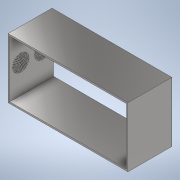
# Autodesk Inventor part: corpo-meio
Saved by Autodesk Inventor 2021 (Build 250183000, 183)
## iProperties
Created: 2023-11-09
Part Number: corpo-meio
Material: Genérico
Document SubType Name: Modeling
Designer: Vinicius
Density: 1 g/cm^3
Appearance: Padrão
Author: Vinicius
Autodesk Inventor part; units mm, degrees
ref_plane "YZ Plane" through (0, 0, 0) normal (1, 0, 0) x (0, 1, 0)
ref_plane "XZ Plane" through (0, 0, 0) normal (0, 1, 0) x (-1, 0, 0)
ref_plane "XY Plane" through (0, 0, 0) normal (0, 0, 1) x (1, 0, 0)
sketch "Esboço2" plane through (0, 0, 0) normal (0, 0, 1) x (1, 0, 0)
  line L0 (-300, -150) -> (300, -150)
  line L1 (300, -150) -> (300, 150)
  line L2 (300, 150) -> (-300, 150)
  line L3 (-300, 150) -> (-300, -150)
  line L4 (-300, -150) -> (300, 150) construction
  line L5 (300, -150) -> (-300, 150) construction
  line L6 (-292, -142) -> (292, -142)
  line L7 (292, -142) -> (292, 142)
  line L8 (292, 142) -> (-292, 142)
  line L9 (-292, 142) -> (-292, -142)
  line L10 (-292, -142) -> (292, 142) construction
  line L11 (292, -142) -> (-292, 142) construction
  point P0 (0, 0)
  dimension "d0" = 300
  dimension "d1" = 600
  dimension "d2" = 584
  dimension "d3" = 284
  constraints: 24 end point, 4 midpoint, 4 parallel, 2 horizontal, 2 perpendicular
  measures "d0" distance of L2.end L0.start
  measures "d1" distance of L1.end L2.end
  measures "d2" distance of L8.end L7.end
  measures "d3" distance of L8.end L6.start
extrude "Extrusão1" add sketch "Esboço2" along normal blind 220
sketch "Esboço3" plane through (-300, -150, 0) normal (-1, 0, 0) x (0, 0, 1)
  line L0 (220, 8) -> (220, 292) projected
  line L1 (0, 0) -> (220, 0) projected
  line L2 (0, 292) -> (220, 292) projected
  line L3 (165, 150) -> (125, 150)
  circle A0 centre (165, 150) radius 1.5
  circle A1 centre (160, 150) radius 1.5
  circle A2 centre (155, 150) radius 1.5
  circle A3 centre (150, 150) radius 1.5
  circle A4 centre (145, 150) radius 1.5
  circle A5 centre (140, 150) radius 1.5
  circle A6 centre (135, 150) radius 1.5
  circle A7 centre (130, 150) radius 1.5
  circle A8 centre (125, 150) radius 1.5
  circle A9 centre (163.4549, 145.2447) radius 1.5
  circle A10 centre (169.0451, 147.0611) radius 1.5
  circle A11 centre (169.0451, 152.9389) radius 1.5
  circle A12 centre (163.4549, 154.7553) radius 1.5
  circle A13 centre (156.9098, 144.1221) radius 1.5
  circle A14 centre (161.9098, 140.4894) radius 1.5
  circle A15 centre (168.0902, 140.4894) radius 1.5
  circle A16 centre (173.0902, 144.1221) radius 1.5
  circle A17 centre (175, 150) radius 1.5
  circle A18 centre (173.0902, 155.8779) radius 1.5
  circle A19 centre (168.0902, 159.5106) radius 1.5
  circle A20 centre (161.9098, 159.5106) radius 1.5
  circle A21 centre (156.9098, 155.8779) radius 1.5
  circle A22 centre (151.2968, 143.899) radius 1.5
  circle A23 centre (154.963, 138.8528) radius 1.5
  circle A24 centre (160.3647, 135.7342) radius 1.5
  circle A25 centre (166.5679, 135.0822) radius 1.5
  circle A26 centre (172.5, 137.0096) radius 1.5
  circle A27 centre (177.1353, 141.1832) radius 1.5
  circle A28 centre (179.6722, 146.8813) radius 1.5
  circle A29 centre (179.6722, 153.1187) radius 1.5
  circle A30 centre (177.1353, 158.8168) radius 1.5
  circle A31 centre (172.5, 162.9904) radius 1.5
  circle A32 centre (166.5679, 164.9178) radius 1.5
  circle A33 centre (160.3647, 164.2658) radius 1.5
  circle A34 centre (154.963, 161.1472) radius 1.5
  circle A35 centre (151.2968, 156.101) radius 1.5
  circle A36 centre (145.9789, 143.8197) radius 1.5
  circle A37 centre (148.8197, 138.2443) radius 1.5
  circle A38 centre (153.2443, 133.8197) radius 1.5
  circle A39 centre (158.8197, 130.9789) radius 1.5
  circle A40 centre (165, 130) radius 1.5
  circle A41 centre (171.1803, 130.9789) radius 1.5
  circle A42 centre (176.7557, 133.8197) radius 1.5
  circle A43 centre (181.1803, 138.2443) radius 1.5
  circle A44 centre (184.0211, 143.8197) radius 1.5
  circle A45 centre (185, 150) radius 1.5
  circle A46 centre (184.0211, 156.1803) radius 1.5
  circle A47 centre (181.1803, 161.7557) radius 1.5
  circle A48 centre (176.7557, 166.1803) radius 1.5
  circle A49 centre (171.1803, 169.0211) radius 1.5
  circle A50 centre (165, 170) radius 1.5
  circle A51 centre (158.8197, 169.0211) radius 1.5
  circle A52 centre (153.2443, 166.1803) radius 1.5
  circle A53 centre (148.8197, 161.7557) radius 1.5
  circle A54 centre (145.9789, 156.1803) radius 1.5
  circle A55 centre (140.7854, 143.7828) radius 1.5
  circle A56 centre (143.0923, 137.9562) radius 1.5
  circle A57 centre (146.7758, 132.8863) radius 1.5
  circle A58 centre (151.6043, 128.8918) radius 1.5
  circle A59 centre (157.2746, 126.2236) radius 1.5
  circle A60 centre (163.4302, 125.0493) radius 1.5
  circle A61 centre (169.6845, 125.4428) radius 1.5
  circle A62 centre (175.6445, 127.3793) radius 1.5
  circle A63 centre (180.9356, 130.7372) radius 1.5
  circle A64 centre (185.2254, 135.3054) radius 1.5
  circle A65 centre (188.2444, 140.7969) radius 1.5
  circle A66 centre (189.8029, 146.8667) radius 1.5
  circle A67 centre (189.8029, 153.1333) radius 1.5
  circle A68 centre (188.2444, 159.2031) radius 1.5
  circle A69 centre (185.2254, 164.6946) radius 1.5
  circle A70 centre (180.9356, 169.2628) radius 1.5
  circle A71 centre (175.6445, 172.6207) radius 1.5
  circle A72 centre (169.6845, 174.5572) radius 1.5
  circle A73 centre (163.4302, 174.9507) radius 1.5
  circle A74 centre (157.2746, 173.7764) radius 1.5
  circle A75 centre (151.6043, 171.1082) radius 1.5
  circle A76 centre (146.7758, 167.1137) radius 1.5
  circle A77 centre (143.0923, 162.0438) radius 1.5
  circle A78 centre (140.7854, 156.2172) radius 1.5
  circle A79 centre (135.6556, 143.7626) radius 1.5
  circle A80 centre (137.5936, 137.7979) radius 1.5
  circle A81 centre (140.7295, 132.3664) radius 1.5
  circle A82 centre (144.9261, 127.7057) radius 1.5
  circle A83 centre (150, 124.0192) radius 1.5
  circle A84 centre (155.7295, 121.4683) radius 1.5
  circle A85 centre (161.8641, 120.1643) radius 1.5
  circle A86 centre (168.1359, 120.1643) radius 1.5
  circle A87 centre (174.2705, 121.4683) radius 1.5
  circle A88 centre (180, 124.0192) radius 1.5
  circle A89 centre (185.0739, 127.7057) radius 1.5
  circle A90 centre (189.2705, 132.3664) radius 1.5
  circle A91 centre (192.4064, 137.7979) radius 1.5
  circle A92 centre (194.3444, 143.7626) radius 1.5
  circle A93 centre (195, 150) radius 1.5
  circle A94 centre (194.3444, 156.2374) radius 1.5
  circle A95 centre (192.4064, 162.2021) radius 1.5
  circle A96 centre (189.2705, 167.6336) radius 1.5
  circle A97 centre (185.0739, 172.2943) radius 1.5
  circle A98 centre (180, 175.9808) radius 1.5
  circle A99 centre (174.2705, 178.5317) radius 1.5
  circle A100 centre (168.1359, 179.8357) radius 1.5
  circle A101 centre (161.8641, 179.8357) radius 1.5
  circle A102 centre (155.7295, 178.5317) radius 1.5
  circle A103 centre (150, 175.9808) radius 1.5
  circle A104 centre (144.9261, 172.2943) radius 1.5
  circle A105 centre (140.7295, 167.6336) radius 1.5
  circle A106 centre (137.5936, 162.2021) radius 1.5
  circle A107 centre (135.6556, 156.2374) radius 1.5
  circle A108 centre (130.5625, 143.7505) radius 1.5
  circle A109 centre (132.2318, 137.7019) radius 1.5
  circle A110 centre (134.9543, 132.0485) radius 1.5
  circle A111 centre (138.6425, 126.9721) radius 1.5
  circle A112 centre (143.1779, 122.6359) radius 1.5
  circle A113 centre (148.4146, 119.1792) radius 1.5
  circle A114 centre (154.1844, 116.713) radius 1.5
  circle A115 centre (160.3018, 115.3168) radius 1.5
  circle A116 centre (166.5703, 115.0352) radius 1.5
  circle A117 centre (172.7882, 115.8775) radius 1.5
  circle A118 centre (178.7559, 117.8165) radius 1.5
  circle A119 centre (184.2814, 120.7899) radius 1.5
  circle A120 centre (189.1872, 124.7022) radius 1.5
  circle A121 centre (193.3156, 129.4275) radius 1.5
  circle A122 centre (196.5339, 134.8141) radius 1.5
  circle A123 centre (198.7387, 140.6887) radius 1.5
  circle A124 centre (199.8591, 146.8626) radius 1.5
  circle A125 centre (199.8591, 153.1374) radius 1.5
  circle A126 centre (198.7387, 159.3113) radius 1.5
  circle A127 centre (196.5339, 165.1859) radius 1.5
  circle A128 centre (193.3156, 170.5725) radius 1.5
  circle A129 centre (189.1872, 175.2978) radius 1.5
  circle A130 centre (184.2814, 179.2101) radius 1.5
  circle A131 centre (178.7559, 182.1835) radius 1.5
  circle A132 centre (172.7882, 184.1225) radius 1.5
  circle A133 centre (166.5703, 184.9648) radius 1.5
  circle A134 centre (160.3018, 184.6832) radius 1.5
  circle A135 centre (154.1844, 183.287) radius 1.5
  circle A136 centre (148.4146, 180.8208) radius 1.5
  circle A137 centre (143.1779, 177.3641) radius 1.5
  circle A138 centre (138.6425, 173.0279) radius 1.5
  circle A139 centre (134.9543, 167.9515) radius 1.5
  circle A140 centre (132.2318, 162.2981) radius 1.5
  circle A141 centre (130.5625, 156.2495) radius 1.5
  circle A142 centre (125.4925, 143.7426) radius 1.5
  circle A143 centre (126.9577, 137.6393) radius 1.5
  circle A144 centre (129.3597, 131.8404) radius 1.5
  circle A145 centre (132.6393, 126.4886) radius 1.5
  circle A146 centre (136.7157, 121.7157) radius 1.5
  circle A147 centre (141.4886, 117.6393) radius 1.5
  circle A148 centre (146.8404, 114.3597) radius 1.5
  circle A149 centre (152.6393, 111.9577) radius 1.5
  circle A150 centre (158.7426, 110.4925) radius 1.5
  circle A151 centre (165, 110) radius 1.5
  circle A152 centre (171.2574, 110.4925) radius 1.5
  circle A153 centre (177.3607, 111.9577) radius 1.5
  circle A154 centre (183.1596, 114.3597) radius 1.5
  circle A155 centre (188.5114, 117.6393) radius 1.5
  circle A156 centre (193.2843, 121.7157) radius 1.5
  circle A157 centre (197.3607, 126.4886) radius 1.5
  circle A158 centre (200.6403, 131.8404) radius 1.5
  circle A159 centre (203.0423, 137.6393) radius 1.5
  circle A160 centre (204.5075, 143.7426) radius 1.5
  circle A161 centre (205, 150) radius 1.5
  circle A162 centre (204.5075, 156.2574) radius 1.5
  circle A163 centre (203.0423, 162.3607) radius 1.5
  circle A164 centre (200.6403, 168.1596) radius 1.5
  circle A165 centre (197.3607, 173.5114) radius 1.5
  circle A166 centre (193.2843, 178.2843) radius 1.5
  circle A167 centre (188.5114, 182.3607) radius 1.5
  circle A168 centre (183.1596, 185.6403) radius 1.5
  circle A169 centre (177.3607, 188.0423) radius 1.5
  circle A170 centre (171.2574, 189.5075) radius 1.5
  circle A171 centre (165, 190) radius 1.5
  circle A172 centre (158.7426, 189.5075) radius 1.5
  circle A173 centre (152.6393, 188.0423) radius 1.5
  circle A174 centre (146.8404, 185.6403) radius 1.5
  circle A175 centre (141.4886, 182.3607) radius 1.5
  circle A176 centre (136.7157, 178.2843) radius 1.5
  circle A177 centre (132.6393, 173.5114) radius 1.5
  circle A178 centre (129.3597, 168.1596) radius 1.5
  circle A179 centre (126.9577, 162.3607) radius 1.5
  circle A180 centre (125.4925, 156.2574) radius 1.5
  line L4 (0, 8) -> (0, 292)
  circle A181 centre (55, 150) radius 1.5
  circle A182 centre (60, 150) radius 1.5
  circle A183 centre (65, 150) radius 1.5
  circle A184 centre (70, 150) radius 1.5
  circle A185 centre (75, 150) radius 1.5
  circle A186 centre (80, 150) radius 1.5
  circle A187 centre (85, 150) radius 1.5
  circle A188 centre (90, 150) radius 1.5
  circle A189 centre (95, 150) radius 1.5
  circle A190 centre (56.5451, 145.2447) radius 1.5
  circle A191 centre (50.9549, 147.0611) radius 1.5
  circle A192 centre (50.9549, 152.9389) radius 1.5
  circle A193 centre (56.5451, 154.7553) radius 1.5
  circle A194 centre (63.0902, 144.1221) radius 1.5
  circle A195 centre (58.0902, 140.4894) radius 1.5
  circle A196 centre (51.9098, 140.4894) radius 1.5
  circle A197 centre (46.9098, 144.1221) radius 1.5
  circle A198 centre (45, 150) radius 1.5
  circle A199 centre (46.9098, 155.8779) radius 1.5
  circle A200 centre (51.9098, 159.5106) radius 1.5
  circle A201 centre (58.0902, 159.5106) radius 1.5
  circle A202 centre (63.0902, 155.8779) radius 1.5
  circle A203 centre (68.7032, 143.899) radius 1.5
  circle A204 centre (65.037, 138.8528) radius 1.5
  circle A205 centre (59.6353, 135.7342) radius 1.5
  circle A206 centre (53.4321, 135.0822) radius 1.5
  circle A207 centre (47.5, 137.0096) radius 1.5
  circle A208 centre (42.8647, 141.1832) radius 1.5
  circle A209 centre (40.3278, 146.8813) radius 1.5
  circle A210 centre (40.3278, 153.1187) radius 1.5
  circle A211 centre (42.8647, 158.8168) radius 1.5
  circle A212 centre (47.5, 162.9904) radius 1.5
  circle A213 centre (53.4321, 164.9178) radius 1.5
  circle A214 centre (59.6353, 164.2658) radius 1.5
  circle A215 centre (65.037, 161.1472) radius 1.5
  circle A216 centre (68.7032, 156.101) radius 1.5
  circle A217 centre (74.0211, 143.8197) radius 1.5
  circle A218 centre (71.1803, 138.2443) radius 1.5
  circle A219 centre (66.7557, 133.8197) radius 1.5
  circle A220 centre (61.1803, 130.9789) radius 1.5
  circle A221 centre (55, 130) radius 1.5
  circle A222 centre (48.8197, 130.9789) radius 1.5
  circle A223 centre (43.2443, 133.8197) radius 1.5
  circle A224 centre (38.8197, 138.2443) radius 1.5
  circle A225 centre (35.9789, 143.8197) radius 1.5
  circle A226 centre (35, 150) radius 1.5
  circle A227 centre (35.9789, 156.1803) radius 1.5
  circle A228 centre (38.8197, 161.7557) radius 1.5
  circle A229 centre (43.2443, 166.1803) radius 1.5
  circle A230 centre (48.8197, 169.0211) radius 1.5
  circle A231 centre (55, 170) radius 1.5
  circle A232 centre (61.1803, 169.0211) radius 1.5
  circle A233 centre (66.7557, 166.1803) radius 1.5
  circle A234 centre (71.1803, 161.7557) radius 1.5
  circle A235 centre (74.0211, 156.1803) radius 1.5
  circle A236 centre (79.2146, 143.7828) radius 1.5
  circle A237 centre (76.9077, 137.9562) radius 1.5
  circle A238 centre (73.2242, 132.8863) radius 1.5
  circle A239 centre (68.3957, 128.8918) radius 1.5
  circle A240 centre (62.7254, 126.2236) radius 1.5
  circle A241 centre (56.5698, 125.0493) radius 1.5
  circle A242 centre (50.3155, 125.4428) radius 1.5
  circle A243 centre (44.3555, 127.3793) radius 1.5
  circle A244 centre (39.0644, 130.7372) radius 1.5
  circle A245 centre (34.7746, 135.3054) radius 1.5
  circle A246 centre (31.7556, 140.7969) radius 1.5
  circle A247 centre (30.1971, 146.8667) radius 1.5
  circle A248 centre (30.1971, 153.1333) radius 1.5
  circle A249 centre (31.7556, 159.2031) radius 1.5
  circle A250 centre (34.7746, 164.6946) radius 1.5
  circle A251 centre (39.0644, 169.2628) radius 1.5
  circle A252 centre (44.3555, 172.6207) radius 1.5
  circle A253 centre (50.3155, 174.5572) radius 1.5
  circle A254 centre (56.5698, 174.9507) radius 1.5
  circle A255 centre (62.7254, 173.7764) radius 1.5
  circle A256 centre (68.3957, 171.1082) radius 1.5
  circle A257 centre (73.2242, 167.1137) radius 1.5
  circle A258 centre (76.9077, 162.0438) radius 1.5
  circle A259 centre (79.2146, 156.2172) radius 1.5
  circle A260 centre (84.3444, 143.7626) radius 1.5
  circle A261 centre (82.4064, 137.7979) radius 1.5
  circle A262 centre (79.2705, 132.3664) radius 1.5
  circle A263 centre (75.0739, 127.7057) radius 1.5
  circle A264 centre (70, 124.0192) radius 1.5
  circle A265 centre (64.2705, 121.4683) radius 1.5
  circle A266 centre (58.1359, 120.1643) radius 1.5
  circle A267 centre (51.8641, 120.1643) radius 1.5
  circle A268 centre (45.7295, 121.4683) radius 1.5
  circle A269 centre (40, 124.0192) radius 1.5
  circle A270 centre (34.9261, 127.7057) radius 1.5
  circle A271 centre (30.7295, 132.3664) radius 1.5
  circle A272 centre (27.5936, 137.7979) radius 1.5
  circle A273 centre (25.6556, 143.7626) radius 1.5
  circle A274 centre (25, 150) radius 1.5
  circle A275 centre (25.6556, 156.2374) radius 1.5
  circle A276 centre (27.5936, 162.2021) radius 1.5
  circle A277 centre (30.7295, 167.6336) radius 1.5
  circle A278 centre (34.9261, 172.2943) radius 1.5
  circle A279 centre (40, 175.9808) radius 1.5
  circle A280 centre (45.7295, 178.5317) radius 1.5
  circle A281 centre (51.8641, 179.8357) radius 1.5
  circle A282 centre (58.1359, 179.8357) radius 1.5
  circle A283 centre (64.2705, 178.5317) radius 1.5
  circle A284 centre (70, 175.9808) radius 1.5
  circle A285 centre (75.0739, 172.2943) radius 1.5
  circle A286 centre (79.2705, 167.6336) radius 1.5
  circle A287 centre (82.4064, 162.2021) radius 1.5
  circle A288 centre (84.3444, 156.2374) radius 1.5
  circle A289 centre (89.4375, 143.7505) radius 1.5
  circle A290 centre (87.7682, 137.7019) radius 1.5
  circle A291 centre (85.0457, 132.0485) radius 1.5
  circle A292 centre (81.3575, 126.9721) radius 1.5
  circle A293 centre (76.8221, 122.6359) radius 1.5
  circle A294 centre (71.5854, 119.1792) radius 1.5
  circle A295 centre (65.8156, 116.713) radius 1.5
  circle A296 centre (59.6982, 115.3168) radius 1.5
  circle A297 centre (53.4297, 115.0352) radius 1.5
  circle A298 centre (47.2118, 115.8775) radius 1.5
  circle A299 centre (41.2441, 117.8165) radius 1.5
  circle A300 centre (35.7186, 120.7899) radius 1.5
  circle A301 centre (30.8128, 124.7022) radius 1.5
  circle A302 centre (26.6844, 129.4275) radius 1.5
  circle A303 centre (23.4661, 134.8141) radius 1.5
  circle A304 centre (21.2613, 140.6887) radius 1.5
  circle A305 centre (20.1409, 146.8626) radius 1.5
  circle A306 centre (20.1409, 153.1374) radius 1.5
  circle A307 centre (21.2613, 159.3113) radius 1.5
  circle A308 centre (23.4661, 165.1859) radius 1.5
  circle A309 centre (26.6844, 170.5725) radius 1.5
  circle A310 centre (30.8128, 175.2978) radius 1.5
  circle A311 centre (35.7186, 179.2101) radius 1.5
  circle A312 centre (41.2441, 182.1835) radius 1.5
  circle A313 centre (47.2118, 184.1225) radius 1.5
  circle A314 centre (53.4297, 184.9648) radius 1.5
  circle A315 centre (59.6982, 184.6832) radius 1.5
  circle A316 centre (65.8156, 183.287) radius 1.5
  circle A317 centre (71.5854, 180.8208) radius 1.5
  circle A318 centre (76.8221, 177.3641) radius 1.5
  circle A319 centre (81.3575, 173.0279) radius 1.5
  circle A320 centre (85.0457, 167.9515) radius 1.5
  circle A321 centre (87.7682, 162.2981) radius 1.5
  circle A322 centre (89.4375, 156.2495) radius 1.5
  circle A323 centre (94.5075, 143.7426) radius 1.5
  circle A324 centre (93.0423, 137.6393) radius 1.5
  circle A325 centre (90.6403, 131.8404) radius 1.5
  circle A326 centre (87.3607, 126.4886) radius 1.5
  circle A327 centre (83.2843, 121.7157) radius 1.5
  circle A328 centre (78.5114, 117.6393) radius 1.5
  circle A329 centre (73.1596, 114.3597) radius 1.5
  circle A330 centre (67.3607, 111.9577) radius 1.5
  circle A331 centre (61.2574, 110.4925) radius 1.5
  circle A332 centre (55, 110) radius 1.5
  circle A333 centre (48.7426, 110.4925) radius 1.5
  circle A334 centre (42.6393, 111.9577) radius 1.5
  circle A335 centre (36.8404, 114.3597) radius 1.5
  circle A336 centre (31.4886, 117.6393) radius 1.5
  circle A337 centre (26.7157, 121.7157) radius 1.5
  circle A338 centre (22.6393, 126.4886) radius 1.5
  circle A339 centre (19.3597, 131.8404) radius 1.5
  circle A340 centre (16.9577, 137.6393) radius 1.5
  circle A341 centre (15.4925, 143.7426) radius 1.5
  circle A342 centre (15, 150) radius 1.5
  circle A343 centre (15.4925, 156.2574) radius 1.5
  circle A344 centre (16.9577, 162.3607) radius 1.5
  circle A345 centre (19.3597, 168.1596) radius 1.5
  circle A346 centre (22.6393, 173.5114) radius 1.5
  circle A347 centre (26.7157, 178.2843) radius 1.5
  circle A348 centre (31.4886, 182.3607) radius 1.5
  circle A349 centre (36.8404, 185.6403) radius 1.5
  circle A350 centre (42.6393, 188.0423) radius 1.5
  circle A351 centre (48.7426, 189.5075) radius 1.5
  circle A352 centre (55, 190) radius 1.5
  circle A353 centre (61.2574, 189.5075) radius 1.5
  circle A354 centre (67.3607, 188.0423) radius 1.5
  circle A355 centre (73.1596, 185.6403) radius 1.5
  circle A356 centre (78.5114, 182.3607) radius 1.5
  circle A357 centre (83.2843, 178.2843) radius 1.5
  circle A358 centre (87.3607, 173.5114) radius 1.5
  circle A359 centre (90.6403, 168.1596) radius 1.5
  circle A360 centre (93.0423, 162.3607) radius 1.5
  circle A361 centre (94.5075, 156.2574) radius 1.5
  point P0 (0, 150)
  dimension "d8" = 150
  dimension "d11" = 55
  dimension "d20" = 5
  dimension "d24" = 360
  dimension "d28" = 360
  dimension "d32" = 360
  dimension "d36" = 360
  dimension "d40" = 360
  dimension "d44" = 360
  dimension "d48" = 360
  dimension "d52" = 360
  constraints: 362 centre point, 8 coincident, 4 end point, 2 horizontal, 384 other
  measures "d8" distance from line of L1 L3.start
  measures "d11" distance from line of L0 L3.start
  measures "d20" distance of A0.centre A1.centre
extrude "Extrusão2" cut sketch "Esboço3" against normal blind 10
sketch "Esboço4" plane through (0, 0, 0) normal (0, 0, -1) x (-1, 0, 0)
  line L0 (-250, 146) -> (250, -146) construction
  line L1 (250, 146) -> (-250, -146) construction
  circle A0 centre (250, -146) radius 2
  circle A1 centre (-250, -146) radius 2
  circle A2 centre (-250, 146) radius 2
  circle A3 centre (250, 146) radius 2
  circle A4 centre (0, -146) radius 2
  circle A5 centre (0, 146) radius 2
  point P0 (0, 0)
  dimension "d56" = 500
  dimension "d57" = 292
  dimension "d58" = 4
  dimension "d59" = 4
  dimension "d60" = 4
  dimension "d61" = 4
  dimension "d62" = 4
  dimension "d63" = 4
  constraints: 6 centre point, 4 end point, 2 midpoint, 1 coincident
  measures "d56" distance of L0.end L1.end
  measures "d57" distance of L1.start L0.end
  measures "d58" diameter of A0
  measures "d59" diameter of A1
  measures "d60" diameter of A2
  measures "d61" diameter of A3
  measures "d62" diameter of A4
  measures "d63" diameter of A5
extrude "Extrusão3" cut sketch "Esboço4" against normal blind 30
chamfer "Chanfro1" distance 1 angle 45 6 edges at (-248, -146, 0) (2, -146, 0) (252, -146, 0) (252, 146, 0) (2, 146, 0) (-248, 146, 0)
